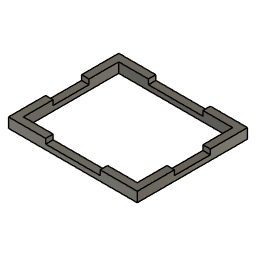
TV stand decoder (Autodesk Fusion 360 design; units mm, degrees)
Autodesk Fusion 360 part; units mm, degrees
sketch "Sketch1" plane through (0, 0, 0) normal (0, 0, 1) x (1, 0, 0)
  line L0 (52, -44.5) -> (-52, -44.5)
  line L1 (-52, -44.5) -> (-52, 44.5)
  line L2 (-52, 44.5) -> (52, 44.5)
  line L3 (52, 44.5) -> (52, -44.5)
  line L4 (52, -44.5) -> (-52, 44.5) construction
  line L5 (-52, -44.5) -> (52, 44.5) construction
  dimension "d1" = 104
  dimension "d2" = 89
  constraint horizontal L0
  constraint perpendicular L0 L1
  constraint parallel L0 L2
  constraint parallel L1 L3
  constraint coincident L4 origin
  constraint coincident L5 origin
  measures "d1" distance of L1 L3
  measures "d2" distance of L0 L2
extrude "Extrude1" add sketch "Sketch1" along normal blind 8
sketch "Sketch4" plane through (0, 0, 8) normal (0, 0, 1) x (1, 0, 0)
  line L0 (46, -38.5) -> (-46, -38.5)
  line L1 (-46, -38.5) -> (-46, 38.5)
  line L2 (-46, 38.5) -> (46, 38.5)
  line L3 (46, 38.5) -> (46, -38.5)
  line L4 (46, -38.5) -> (-46, 38.5) construction
  line L5 (-46, -38.5) -> (46, 38.5) construction
  dimension "d5" = 77
  dimension "d6" = 92
  constraint horizontal L0
  constraint perpendicular L0 L1
  constraint parallel L0 L2
  constraint parallel L1 L3
  constraint coincident L4 origin
  constraint coincident L5 origin
  measures "d5" distance of L0 L2
  measures "d6" distance of L1 L3
extrude "Extrude2" cut sketch "Sketch4" against normal blind 8
sketch "Sketch5" plane through (0, 0, 8) normal (0, 0, 1) x (-1, 0, 0)
  line L0 (46, 38.5) -> (46, -38.5)
  line L1 (46, -38.5) -> (-46, -38.5)
  line L2 (-46, -38.5) -> (-46, 38.5)
  line L3 (-46, 38.5) -> (46, 38.5)
  line L4 (-52, -44.5) -> (52, -44.5)
  line L5 (52, -44.5) -> (52, 44.5)
  line L6 (52, 44.5) -> (-52, 44.5)
  line L7 (-52, 44.5) -> (-52, -44.5)
  line L8 (52, -14.5) -> (46, -14.5)
  line L9 (46, -14.5) -> (46, 14.5)
  line L10 (46, 14.5) -> (52, 14.5)
  line L11 (52, 14.5) -> (52, -14.5)
  dimension "d9" = 29
  dimension "d10" = 6
  constraint horizontal L8
  constraint vertical L9
  constraint horizontal L10
  constraint vertical L11
  constraint coincident L5 L8.start
  measures "d9" distance of L8 L10
  measures "d10" distance of L9 L11
extrude "Extrude3" cut sketch "Sketch5" against normal blind 4 contours L0 L5 L8 L9 L10 L11
sketch "Sketch6" plane through (0, 0, 8) normal (0, 0, 1) x (-1, 0, 0)
  line L0 (46, 14.5) -> (52, 14.5)
  line L1 (52, 14.5) -> (52, 44.5)
  line L2 (52, 44.5) -> (-52, 44.5)
  line L3 (-52, 44.5) -> (-52, -44.5)
  line L4 (-52, -44.5) -> (52, -44.5)
  line L5 (52, -44.5) -> (52, -14.5)
  line L6 (52, -14.5) -> (46, -14.5)
  line L7 (46, -14.5) -> (46, -38.5)
  line L8 (46, -38.5) -> (-46, -38.5)
  line L9 (-46, -38.5) -> (-46, 38.5)
  line L10 (-46, 38.5) -> (46, 38.5)
  line L11 (46, 38.5) -> (46, 14.5)
  line L12 (-46, -14.5) -> (-52, -14.5)
  line L13 (-52, -14.5) -> (-52, 14.5)
  line L14 (-52, 14.5) -> (-46, 14.5)
  line L15 (-46, 14.5) -> (-46, -14.5)
  dimension "d13" = 29
  dimension "d14" = 6
  constraint horizontal L12
  constraint vertical L13
  constraint horizontal L14
  constraint vertical L15
  constraint coincident L9 L12.start
  measures "d13" distance of L12 L14
  measures "d14" distance of L13 L15
extrude "Extrude4" cut sketch "Sketch6" against normal blind 4 contours L3 L9 L12 L13 L14 L15
sketch "Sketch7" plane through (0, 0, 8) normal (0, 0, 1) x (-1, 0, 0)
  line L0 (-46, -14.5) -> (-52, -14.5)
  line L1 (-52, -14.5) -> (-52, -44.5)
  line L2 (-52, -44.5) -> (52, -44.5)
  line L3 (52, -44.5) -> (52, -14.5)
  line L4 (52, -14.5) -> (46, -14.5)
  line L5 (46, -14.5) -> (46, -38.5)
  line L6 (46, -38.5) -> (-46, -38.5)
  line L7 (-46, -38.5) -> (-46, -14.5)
  line L8 (22, -44.5) -> (-22, -44.5)
  line L9 (-22, -44.5) -> (-22, -38.5)
  line L10 (-22, -38.5) -> (22, -38.5)
  line L11 (22, -38.5) -> (22, -44.5)
  dimension "d17" = 6
  dimension "d18" = 44
  constraint horizontal L8
  constraint vertical L9
  constraint horizontal L10
  constraint vertical L11
  constraint coincident L2 L8.start
  measures "d17" distance of L8 L10
  measures "d18" distance of L9 L11
extrude "Extrude5" cut sketch "Sketch7" against normal blind 4 contours L2 L6 L8 L9 L10 L11
sketch "Sketch8" plane through (0, 0, 8) normal (0, 0, 1) x (-1, 0, 0)
  line L0 (-52, 14.5) -> (-46, 14.5)
  line L1 (-46, 14.5) -> (-46, 38.5)
  line L2 (-46, 38.5) -> (46, 38.5)
  line L3 (46, 38.5) -> (46, 14.5)
  line L4 (46, 14.5) -> (52, 14.5)
  line L5 (52, 14.5) -> (52, 44.5)
  line L6 (52, 44.5) -> (-52, 44.5)
  line L7 (-52, 44.5) -> (-52, 14.5)
  line L8 (22.0005, 38.5) -> (-21.9995, 38.5)
  line L9 (-21.9995, 38.5) -> (-21.9995, 44.5)
  line L10 (-21.9995, 44.5) -> (22.0005, 44.5)
  line L11 (22.0005, 44.5) -> (22.0005, 38.5)
  dimension "d21" = 44
  dimension "d22" = 6
  constraint horizontal L8
  constraint vertical L9
  constraint horizontal L10
  constraint vertical L11
  constraint coincident L2 L8.start
  measures "d21" distance of L9 L11
  measures "d22" distance of L8 L10
extrude "Extrude6" cut sketch "Sketch8" against normal blind 4 contours L2 L6 L8 L9 L10 L11
